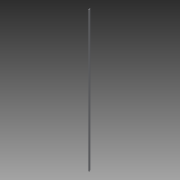
# Autodesk Inventor part: Cornière
Saved by Autodesk Inventor 2015 SP1 (Build 190203100, 203)
## iProperties
Created: 2015-04-17
Part Number: Cornière
Material: Generic
Document SubType Name: Modeling
Designer: Cyril
Density: 1 g/cm^3
Appearance: Default
Author: Cyril
Autodesk Inventor part; units mm, degrees
ref_plane "YZ Plane" through (0, 0, 0) normal (1, 0, 0) x (0, 1, 0)
ref_plane "XZ Plane" through (0, 0, 0) normal (0, 1, 0) x (-1, 0, 0)
ref_plane "XY Plane" through (0, 0, 0) normal (0, 0, 1) x (1, 0, 0)
sketch "Sketch1" plane through (0, 0, 0) normal (0, 0, 1) x (1, 0, 0)
  line L0 (0, 0) -> (0, 30)
  arc A0 (5, 25) -> (0, 30) centre (0, 25) ccw
  line L1 (5, 25) -> (5, 10)
  arc A1 (5, 10) -> (10, 5) centre (10, 10) ccw
  line L2 (10, 5) -> (15, 5)
  arc A2 (20, 0) -> (15, 5) centre (15, 0) ccw
  line L3 (20, 0) -> (20, 0)
  line L4 (20, 0) -> (0, 0)
  dimension "d1" = 30
  dimension "d2" = 5
  dimension "d3" = 20
  dimension "d4" = 5
  dimension "d5" = 5
  constraints: 10 end point, 7 point on circle, 5 tangent, 3 centre point, 2 perpendicular, 1 horizontal, 1 parallel, 1 point on line, 1 vertical
  measures "d1" distance of L0.start L0.end
  measures "d2" distance between parallel lines of L1 L0
  measures "d3" distance of L3.end L0.start
  measures "d4" distance between parallel lines of L4 L2
  measures "d5" radius of A1
extrude "Extrusion1" add sketch "Sketch1" along normal mid plane 2000
body "Solid1"
